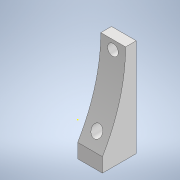
# Autodesk Inventor part: ENCODERV2PLATE
Saved by Autodesk Inventor 2022 (Build 260153070, 153G)
## iProperties
Created: 2022-02-01
Part Number: ENCODERV2PLATE
Material: Generic
Document SubType Name: Modeling
Designer: a laptop
Density: 1 g/cm^3
Appearance: Default
Author: a laptop
Autodesk Inventor part; units mm, degrees
ref_plane "YZ Plane" through (0, 0, 0) normal (1, 0, 0) x (0, 1, 0)
ref_plane "XZ Plane" through (0, 0, 0) normal (0, 1, 0) x (-1, 0, 0)
ref_plane "XY Plane" through (0, 0, 0) normal (0, 0, 1) x (1, 0, 0)
sketch "Sketch1" plane through (0, 0, 0) normal (0, 0, 1) x (1, 0, 0)
  circle A0 centre (13, 8.75) radius 1.5 projected
  circle A1 centre (13, -8.75) radius 1.5 projected
  line L0 (9.525, 11.15) -> (16.475, 11.15)
  line L1 (16.475, 11.15) -> (16.475, -16.3)
  line L2 (9.525, 11.15) -> (9.525, -16.3)
  line L3 (9.525, -16.3) -> (16.475, -16.3)
  point P0 (0, 0)
  dimension "d0" = 27.45
  dimension "d1" = 3.475
  dimension "d2" = 2.4
  dimension "d3" = 3.475
  constraints: 8 end point, 2 horizontal, 1 parallel, 1 perpendicular, 1 vertical
  measures "d0" distance of L0.end L1.end
  measures "d1" distance from line of L2 A0.centre
  measures "d2" distance from line of A0.centre L0
  measures "d3" distance from line of L1 A0.centre
extrude "Extrusion1" add sketch "Sketch1" along normal blind 9.5
sketch "Sketch2" plane through (9.525, -16.3, 0) normal (-1, 0, 0) x (0, 0, 1)
  line L0 (0, 27.45) -> (9.5, 27.45) projected
  line L1 (9.5, 0) -> (9.5, 27.45) projected
  arc A0 (3, 27.45) -> (9.5, 4) centre (48.5502, 27.45) ccw
  line L2 (0, 27.45) -> (9.5, 27.45) projected
  point P0 (0, 16.3)
  dimension "d6" = 3
  dimension "d7" = 4
  constraints: 2 point on circle, 2 point on line, 1 centre point, 1 line through centre
  measures "d6" distance of L0.start A0.start
  measures "d7" distance of L1.start A0.end
extrude "Extrusion2" cut sketch "Sketch2" against normal blind 10
sketch "Sketch3" plane through (9.525, -16.3, 0) normal (0, -1, 0) x (1, 0, 0)
  line L0 (0, 0) -> (0, 9.5) projected
  line L1 (0, 0) -> (6.95, 0) projected
  line L2 (0, 4.75) -> (6.95, 4.75)
  line L3 (6.95, 4.75) -> (6.95, 0)
  line L4 (6.95, 0) -> (0, 0)
  line L5 (0, 0) -> (0, 4.75)
  circle A0 centre (3.855, 7.075) radius 1.375
  point P0 (-9.525, 0)
  dimension "d14" = 3.855
  dimension "d15" = 2.325
  dimension "d16" = 2.75
  constraints: 8 end point, 2 parallel, 1 centre point, 1 horizontal, 1 midpoint, 1 perpendicular
  measures "d14" distance from line of L0 A0.centre
  measures "d15" distance from line of L2 A0.centre
  measures "d16" diameter of A0
extrude "Extrusion3" cut sketch "Sketch3" against normal blind 7.9125 contours A0
extrude "Extrusion4" cut sketch "Sketch3" against normal blind 1.25 contours L0 L2 L3 L1
sketch "Sketch4" plane through (0, 0, 9.5) normal (0, 0, 1) x (1, 0, 0)
  circle A0 centre (13, -8.75) radius 3.25
  circle A1 centre (13, 8.75) radius 3.25
  circle A2 centre (13, -8.75) radius 1.5 projected
  circle A3 centre (13, 8.75) radius 1.5 projected
  point P0 (0, 0)
  dimension "d17" = 6.5
  constraints: 2 centre point, 2 concentric, 1 equal radius
  measures "d17" diameter of A0
extrude "Extrusion5" cut sketch "Sketch4" against normal blind 4.7875 contours A0
extrude "Extrusion6" cut sketch "Sketch4" against normal up to surface (6.5 mm away) contours A1 | A3
body "Solid1"
